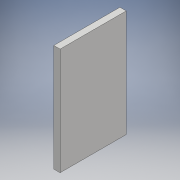
# Autodesk Inventor part: Rear Wall
Saved by Autodesk Inventor 2017 (Build 210142000, 142)
## iProperties
Created: 2017-11-21
Part Number: Rear Wall
Material: Generic
Document SubType Name: Modeling
Designer: Shlomee
Density: 1 g/cm^3
Appearance: Default
Author: Shlomee
Autodesk Inventor part; units mm, degrees
ref_plane "YZ Plane" through (0, 0, 0) normal (1, 0, 0) x (0, 1, 0)
ref_plane "XZ Plane" through (0, 0, 0) normal (0, 1, 0) x (-1, 0, 0)
ref_plane "XY Plane" through (0, 0, 0) normal (0, 0, 1) x (1, 0, 0)
sketch "Sketch3" plane through (0, 0, 0) normal (1, 0, 0) x (0, 1, 0)
  line L0 (12.4424, 18.542) -> (-8.5576, 18.542)
  line L1 (-8.5576, 18.542) -> (-8.5576, -15.458)
  line L2 (-8.5576, -15.458) -> (12.4424, -15.458)
  line L3 (12.4424, -15.458) -> (12.4424, 18.542)
  point P0 (0, 0)
  dimension "d4" = 21
  dimension "d5" = 34
  constraints: 8 end point, 2 parallel, 1 horizontal, 1 perpendicular
  measures "d4" distance of L1.end L2.end
  measures "d5" distance of L2.end L0.start
extrude "Extrusion2" add sketch "Sketch3" along normal blind 2
body "Solid2"
